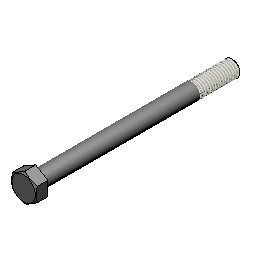
COTS 4 Post Jig v1.00 (Autodesk Fusion 360 archive; units mm, degrees)
design "Hex Bolt ASME B18.2.1 - 1/2-13 UNC x 6 Steel Grade 2 Plain"
description: Hex Bolt ASME B18.2.1 - 1/2-13 UNC x 6
part number: HB ASME B18.2.1 - 1/2-13 UNC x 6 Steel Grade 2 Plain
Autodesk Fusion 360 part; units mm, degrees
sketch "Sketch1" plane through (0, 0, 0) normal (0, 1, 0) x (1, 0, 0)
  line L0 (-6.35, 0) -> (-6.35, 152.4)
  line L1 (-6.35, 152.4) -> (0, 152.4)
  line L2 (0, 152.4) -> (0, -9.2456)
  line L3 (-6.35, 0) -> (-11.0014, 0)
  line L4 (-11.0014, 0) -> (-11.0014, -8.1183)
  line L5 (-9.0487, -9.2456) -> (0, -9.2456)
  line L6 (-11.0014, -8.1183) -> (-9.0487, -9.2456)
  dimension "d81" = 22.0028
  dimension "d135" = 12.7
  dimension "d148" = 9.2456
  dimension "d149" = 152.4
  dimension "d170" = 18.0975
  dimension "d171" = 30
  constraint perpendicular L0 L1
  constraint perpendicular L0 L3
  constraint coincident origin L3
  constraint vertical L0
  constraint vertical L2
  constraint parallel L2 L4
  constraint coincident L2 L5.end
  constraint perpendicular L2 L5
  constraint coincident L0.start L3.start
  constraint coincident L0.end L1.start
  constraint coincident origin L2
  measures "d148" distance of L3 L5
  measures "d149" distance of L1 L3
  measures "d171" angle of L5 L6
revolve "Revolve1" add sketch "Sketch1" angle 360 about axis through (0, 0, -152.4) along (0, 0, 1)
sketch "Sketch8" plane through (0, 0, 9.2456) normal (0, 0, 1) x (1, 0, 0)
  line L0 (0, 0) -> (-9.525, 0) construction
  line L1 (-9.525, -5.505) -> (-9.525, 5.505)
  circle A0 centre (0, 0) radius 11.0014
  dimension "d114" = 9.525
  constraint coincident L0.start A0.centre
  constraint horizontal L0
  constraint perpendicular L0 L1
  constraint coincident L1.end A0
  constraint coincident L0.end L1
  constraint coincident L1.start A0
  measures "d114" distance of L0.start L1
extrude "Extrude5" cut sketch "Sketch8" against normal blind 9.2456 contours L1 A0 picked at (-9.7632, -1.3408)
pattern_circular "C-Pattern2" count 6 over 360 about axis through (0, 0, 1.75) along (0, 0, 1) of "Extrude5"
fillet "Fillet7" radius 0.762 1 edges at (-5.9203, 2.2963, 0)
thread "Thread3" "ANSI Unified Screw Threads 0.5 1/2-13 UNC 1/2-13 UNC 2A" major diameter 12.5247 minor diameter 10.3353 pitch 1.9538 angle 60 resizes the face on face at (-6.3421, 0.3165, -51.308) from (0, 0, -120.65) to (0, 0, -152.4)
sketch "Sketch13" plane through (0, 0, 0) normal (0, 1, 0) x (1, 0, 0)
  line L0 (0, 152.4) -> (0, -9.2456)
  line L1 (0, 152.4) -> (-6.477, 152.4)
  line L2 (-6.477, 152.4) -> (-6.477, 151.2014)
  line L3 (-6.477, 151.2014) -> (-5.1514, 152.4)
  dimension "d172" = 1.1986
  dimension "d173" = 5.1514
  dimension "d174" = 6.477
  constraint coincident L0.start L1.start
  constraint perpendicular L0 L1
  constraint perpendicular L1 L2
  constraint coincident L1 L3.end
  measures "d172" distance of L1 L2.end
  measures "d173" distance of L0 L3.end
  measures "d174" distance of L0.start L2
revolve "Revolve4" cut sketch "Sketch13" angle 360 about axis through (0, 0, 1.75) along (0, 0, 1)
equation "d81 = adsk_headdia"
equation "d89 = -adsk_headh"
equation "d114 = adsk_waflat / 2"
equation "d135 = adsk_nomdia"
equation "adsk_nomlen = 6.00 in"
equation "adsk_headh = 0.364 in"
equation "adsk_headdia = 0.86625 in"
equation "adsk_nomdia = 0.50 in"
equation "adsk_waflat = 0.75 in"
equation "adsk_thrlen = 1.25 in"
equation "adsk_midfillet = 0.03 in"
equation "d148 = adsk_headh"
equation "d149 = adsk_nomlen"
equation "d151 = adsk_midfillet"
equation "adsk_endpointdia = 0.405623 in"
equation "adsk_startlen = 0.047188 in"
equation "d170 = adsk_waflat * 0.95"
equation "d172 = adsk_startlen"
equation "d173 = adsk_endpointdia / 2"
equation "d174 = adsk_nomdia * 0.51"
equation "d176 = min(adsk_thrlen; adsk_nomlen - adsk_midfillet - 0.001 in)"

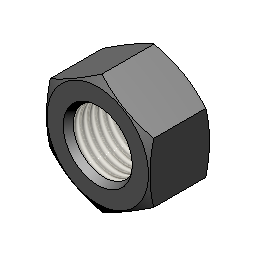
design "Hex Nut ASME B18.2.2 - 3/8-24 Steel Grade 2H Plain"
description: Hex Nut ASME B18.2.2 - 3/8-24
part number: HN ASME B18.2.2 - 3/8-24 Steel Grade 2H Plain
Autodesk Fusion 360 part; units mm, degrees
sketch "Sketch1" plane through (0, 0, 0) normal (0, 1, 0) x (1, 0, 0)
  line L0 (0, 0) -> (0, -8.3566)
  line L1 (-4.7625, 0) -> (-7.0071, 0)
  line L2 (-7.0071, 0) -> (-8.2584, -0.5835)
  line L3 (-8.2584, -0.5835) -> (-8.2584, -7.7731)
  line L4 (-8.2584, -7.7731) -> (-7.0071, -8.3566)
  line L5 (-7.0071, -8.3566) -> (-4.7625, -8.3566)
  line L6 (-4.7625, -8.3566) -> (-4.7625, 0)
  line L7 (-7.0071, -8.3566) -> (-7.0071, 0) construction
  dimension "d121" = 9.525
  dimension "d122" = 25
  dimension "d123" = 25
  dimension "d128" = 16.5167
  dimension "d170" = 14.0142
  dimension "d176" = 8.3566
  constraint vertical L0
  constraint coincident L0 L0.end
  constraint coincident origin L0
  constraint horizontal L1
  constraint perpendicular L1 L3
  constraint perpendicular L3 L5
  constraint perpendicular L5 L6
  constraint coincident L0.start L1
  constraint coincident L0.end L5
  constraint coincident L0.start origin
  constraint vertical L7
  measures "d122" angle of L1 L2
  measures "d123" angle of L4 L5
  measures "d176" distance of L1.start L5
revolve "Revolve1" add sketch "Sketch1" angle 360 about axis through (0, 0, 0) along (0, 0, 1)
sketch "Sketch8" plane through (0, 0, 8.3566) normal (0, 0, 1) x (1, 0, 0)
  line L0 (0, 0) -> (-14.3002, 0) construction
  line L1 (-7.1501, -4.1324) -> (-7.1501, 4.1324)
  circle A0 centre (0, 0) radius 4.7625
  circle A1 centre (0, 0) radius 8.2584
  dimension "d114" = 7.1501
  constraint horizontal L0
  constraint perpendicular L0 L1
  constraint midpoint L0 L1
  constraint coincident L0.start A0.centre
  constraint coincident L1.end A1
  measures "d114" distance of L0.start L1
extrude "Extrude5" cut sketch "Sketch8" against normal blind 8.3566 contours L1 A1 picked at (-7.3289, 1.0065)
pattern_circular "C-Pattern2" count 6 over 360 about axis through (0, 0, 1.75) along (0, 0, 1) of "Extrude5"
thread "Thread3" "ANSI Unified Screw Threads 0.375 3/8-24 UNF 3/8-24 UNF 2B" major diameter 9.525 minor diameter 8.509 pitch 1.0583 angle 60 resizes the face on face at (-4.7388, 0.4742, 2.7855)
sketch "Sketch12" plane through (0, 0, 0) normal (0, 1, 0) x (1, 0, 0)
  line L0 (0, 0) -> (-4.7625, 0)
  line L1 (0, 0) -> (0, -8.3566)
  line L2 (0, -8.3566) -> (-4.7625, -8.3566)
  line L3 (-4.7625, -8.3566) -> (-2.3502, -4.1783)
  line L4 (-4.7625, 0) -> (-2.3502, -4.1783)
  dimension "d164" = 60
  dimension "d165" = 60
  dimension "d175" = 4.7625
  constraint coincident L0.start L1.start
  constraint horizontal L0
  constraint coincident L1.end L2.start
  constraint perpendicular L1 L2
  constraint vertical L0.end L2.end
  constraint coincident L3.end L4.end
  measures "d164" angle of L0 L4
  measures "d165" angle of L2 L3
  measures "d175" distance of L0.end L1
revolve "Revolve3" cut sketch "Sketch12" angle 360 about axis through (0, 0, 1.75) along (0, 0, 1)
equation "d89 = -adsk_nheig"
equation "d114 = adsk_waflat / 2"
equation "adsk_chamang1 = 25.00 deg"
equation "adsk_chamang2 = 25.00 deg"
equation "d121 = adsk_nomdia"
equation "d122 = adsk_chamang1"
equation "d123 = adsk_chamang2"
equation "d128 = adsk_maxdia"
equation "adsk_nheig = 0.329 in"
equation "adsk_maxdia = 0.650265 in"
equation "adsk_nomdia = 0.375 in"
equation "adsk_waflat = 0.563 in"
equation "d162 = adsk_nheig"
equation "adsk_beardia = adsk_waflat * 0.98"
equation "d170 = adsk_beardia"
equation "d175 = adsk_nomdia * 0.50"
equation "d176 = adsk_nheig"

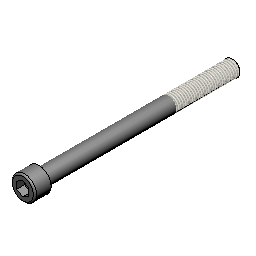
design "Hexagon Socket Head Cap Screw ANSI B18.3 - 1/4-28 UNF x 3 Steel Grade 2 Plain"
description: Hexagon Socket Head Cap Screw ANSI B18.3 - 1/4-28 UNF x 3
part number: HSHCS ANSI B18.3 - 1/4-28 UNF x 3 Steel Grade 2 Plain
Autodesk Fusion 360 part; units mm, degrees
sketch "Sketch1" plane through (0, 0, 0) normal (0, 1, 0) x (1, 0, 0)
  line L0 (-3.175, 0) -> (-3.175, 76.2)
  line L1 (-3.175, 76.2) -> (0, 76.2)
  line L2 (0, 76.2) -> (0, -6.35)
  line L3 (-3.175, 0) -> (-4.7625, 0)
  line L4 (-4.7625, 0) -> (-4.7625, -6.35)
  line L5 (-4.7625, -6.35) -> (0, -6.35)
  dimension "d9" = 6.35
  dimension "d66" = 9.525
  dimension "d107" = 6.35
  dimension "d108" = 76.2
  constraint perpendicular L0 L1
  constraint collinear origin L1.end L2.end
  constraint perpendicular L0 L3
  constraint coincident origin L3
  constraint vertical L0
  constraint vertical L2
  constraint parallel L2 L4
  constraint coincident L2 L5.end
  constraint perpendicular L2 L5
  measures "d107" distance of L3.end L5
  measures "d108" distance of origin L1
revolve "Revolve1" add sketch "Sketch1" angle 360 about axis through (0, 0, -76.2) along (0, 0, 1)
ref_plane "WorkPlane1" through (0, 0, 6.35) normal (0, 0, 1) x (1, 0, 0)
sketch "Sketch6" plane through (0, 0, 6.35) normal (0, 0, 1) x (1, 0, 0)
  line L0 (-2.3876, 0) -> (2.3876, 0) construction
  line L1 (0, 0) -> (-2.3876, 1.3785)
  line L2 (-2.3876, -1.3785) -> (-2.3876, 1.3785)
  line L3 (-2.3876, -1.3785) -> (0, 0)
  dimension "d106" = 150
  dimension "d109" = 4.7752
  constraint horizontal L0
  constraint midpoint L1.start L0
  constraint coincident L1.start L3.end
  constraint perpendicular L0 L2
  constraint midpoint L0.start L2
  constraint coincident L1.end L2.end
  measures "d106" angle of L0 L1
  measures "d109" distance of L0.end L2
extrude "Extrude1" cut sketch "Sketch6" against normal blind 3.048
pattern_circular "C-Pattern1" count 6 over 360 about axis through (0, 0, 1.75) along (0, 0, 1) of "Extrude1"
extrude "Extrude2" cut 1 faces at (0.7959, 0.4595, 3.302) along direction (0, 0, -1) blind 3.048 draft -85
thread "Thread3" "ANSI Unified Screw Threads 0.25 1/4-28 UNF 1/4-28 UNF 2A" major diameter 6.2433 minor diameter 5.2426 pitch 0.9071 angle 60 resizes the face on face at (-3.1711, 0.1583, -50.8) from (0, 0, -50.8) to (0, 0, -76.2)
fillet "Fillet4" radius 0.635 1 edges at (-4.4402, 1.7222, 6.35)
sketch "Sketch7" plane through (0, 0, 0) normal (0, 1, 0) x (1, 0, 0)
  line L0 (-3.2385, 76.2) -> (-3.2385, 75.659)
  line L1 (-3.2385, 75.659) -> (-2.634, 76.2)
  line L2 (0, 76.2) -> (0, -6.35)
  line L3 (-3.2385, 76.2) -> (0, 76.2)
  dimension "d103" = 3.2385
  dimension "d110" = 2.634
  dimension "d111" = 0.541
  constraint coincident L2.start L3.end
  constraint perpendicular L2 L3
  constraint coincident L1.end L3
  constraint perpendicular L0 L3
  measures "d103" distance of origin L0
  measures "d110" distance of L1.end L2
  measures "d111" distance of L0.end L3
revolve "Revolve3" cut sketch "Sketch7" angle 360 about axis through (0, 0, 1.75) along (0, 0, 1)
equation "d9 = adsk_nomdia"
equation "d31 = -adsk_phildepth"
equation "d66 = adsk_headdia"
equation "d71 = adsk_headh"
equation "d76 = -adsk_phildepth"
equation "adsk_nomlen = 3.00 in"
equation "adsk_headh = 0.25 in"
equation "adsk_headdia = 0.375 in"
equation "adsk_nomdia = 0.25 in"
equation "adsk_philwidth = 0.188 in"
equation "adsk_phildepth = 0.12 in"
equation "adsk_thrlen = 1.00 in"
equation "d93 = adsk_nomdia * 0.1"
equation "adsk_startlen = 0.0213 in"
equation "adsk_endpointdia = 0.2074 in"
equation "d103 = adsk_nomdia * 0.51"
equation "d107 = adsk_headh"
equation "d108 = adsk_nomlen"
equation "d109 = adsk_philwidth"
equation "d110 = adsk_endpointdia / 2"
equation "d111 = adsk_startlen"
equation "d113 = min(adsk_thrlen; adsk_nomlen - 0.001 mm)"

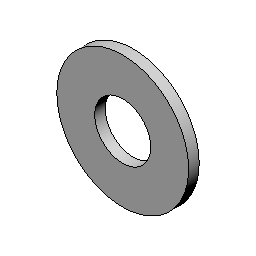
design "Plain Washer ASME B18.21.1 - 1/2 - Regular - Type B Steel 100 HV Zinc"
description: Plain Washer ASME B18.21.1 - 1/2 - Regular - Type B
part number: PW ASME B18.21.1 - 1/2 - BR Steel 100 HV Zinc
Autodesk Fusion 360 part; units mm, degrees
sketch "Sketch1" plane through (0, 0, 0) normal (0, 0, 1) x (1, 0, 0)
  circle A0 centre (0, 0) radius 15.875
  circle A1 centre (0, 0) radius 6.7437
  dimension "d4" = 31.75
  dimension "d5" = 13.4874
  constraint coincident A0.centre A1.centre
  measures "d4" diameter of A0
  measures "d5" diameter of A1
extrude "Extrude2" add sketch "Sketch1" along normal blind 2.54
equation "d4 = adsk_woutdia"
equation "d5 = adsk_windia"
equation "adsk_woutdia = 1.25 in"
equation "adsk_windia = 0.531 in"
equation "adsk_wthick = 0.10 in"
equation "d20 = adsk_wthick"
equation "d41 = adsk_wthick"

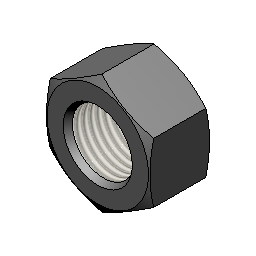
design "Hex Nut ASME B18.2.2 - 1/2-20 Steel Grade 2H Plain"
description: Hex Nut ASME B18.2.2 - 1/2-20
part number: HN ASME B18.2.2 - 1/2-20 Steel Grade 2H Plain
Autodesk Fusion 360 part; units mm, degrees
sketch "Sketch1" plane through (0, 0, 0) normal (0, 1, 0) x (1, 0, 0)
  line L0 (0, 0) -> (0, -11.1252)
  line L1 (-6.35, 0) -> (-9.3345, 0)
  line L2 (-9.3345, 0) -> (-11.0014, -0.7773)
  line L3 (-11.0014, -0.7773) -> (-11.0014, -10.3479)
  line L4 (-11.0014, -10.3479) -> (-9.3345, -11.1252)
  line L5 (-9.3345, -11.1252) -> (-6.35, -11.1252)
  line L6 (-6.35, -11.1252) -> (-6.35, 0)
  line L7 (-9.3345, -11.1252) -> (-9.3345, 0) construction
  dimension "d121" = 12.7
  dimension "d122" = 25
  dimension "d123" = 25
  dimension "d128" = 22.0028
  dimension "d170" = 18.669
  dimension "d176" = 11.1252
  constraint vertical L0
  constraint coincident L0 L0.end
  constraint coincident origin L0
  constraint horizontal L1
  constraint perpendicular L1 L3
  constraint perpendicular L3 L5
  constraint perpendicular L5 L6
  constraint coincident L0.start L1
  constraint coincident L0.end L5
  constraint coincident L0.start origin
  constraint vertical L7
  measures "d122" angle of L1 L2
  measures "d123" angle of L4 L5
  measures "d176" distance of L1.start L5
revolve "Revolve1" add sketch "Sketch1" angle 360 about axis through (0, 0, 0) along (0, 0, 1)
sketch "Sketch8" plane through (0, 0, 11.1252) normal (0, 0, 1) x (1, 0, 0)
  line L0 (0, 0) -> (-19.05, 0) construction
  line L1 (-9.525, -5.505) -> (-9.525, 5.505)
  circle A0 centre (0, 0) radius 6.35
  circle A1 centre (0, 0) radius 11.0014
  dimension "d114" = 9.525
  constraint horizontal L0
  constraint perpendicular L0 L1
  constraint midpoint L0 L1
  constraint coincident L0.start A0.centre
  constraint coincident L1.end A1
  measures "d114" distance of L0.start L1
extrude "Extrude5" cut sketch "Sketch8" against normal blind 11.1252 contours L1 A1 picked at (-9.7632, 1.3408)
pattern_circular "C-Pattern2" count 6 over 360 about axis through (0, 0, 1.75) along (0, 0, 1) of "Extrude5"
thread "Thread3" "ANSI Unified Screw Threads 0.5 1/2-20 UNF 1/2-20 UNF 2B" major diameter 12.7 minor diameter 11.4681 pitch 1.27 angle 60 resizes the face on face at (-6.3421, 0.3165, 7.4168)
sketch "Sketch12" plane through (0, 0, 0) normal (0, 1, 0) x (1, 0, 0)
  line L0 (0, 0) -> (-6.35, 0)
  line L1 (0, 0) -> (0, -11.1252)
  line L2 (0, -11.1252) -> (-6.35, -11.1252)
  line L3 (-6.35, -11.1252) -> (-3.1384, -5.5626)
  line L4 (-6.35, 0) -> (-3.1384, -5.5626)
  dimension "d164" = 60
  dimension "d165" = 60
  dimension "d175" = 6.35
  constraint coincident L0.start L1.start
  constraint horizontal L0
  constraint coincident L1.end L2.start
  constraint perpendicular L1 L2
  constraint vertical L0.end L2.end
  constraint coincident L3.end L4.end
  measures "d164" angle of L0 L4
  measures "d165" angle of L2 L3
  measures "d175" distance of L0.end L1
revolve "Revolve3" cut sketch "Sketch12" angle 360 about axis through (0, 0, 1.75) along (0, 0, 1)
equation "d89 = -adsk_nheig"
equation "d114 = adsk_waflat / 2"
equation "adsk_chamang1 = 25.00 deg"
equation "adsk_chamang2 = 25.00 deg"
equation "d121 = adsk_nomdia"
equation "d122 = adsk_chamang1"
equation "d123 = adsk_chamang2"
equation "d128 = adsk_maxdia"
equation "adsk_nheig = 0.438 in"
equation "adsk_maxdia = 0.86625 in"
equation "adsk_nomdia = 0.50 in"
equation "adsk_waflat = 0.75 in"
equation "d162 = adsk_nheig"
equation "adsk_beardia = adsk_waflat * 0.98"
equation "d170 = adsk_beardia"
equation "d175 = adsk_nomdia * 0.50"
equation "d176 = adsk_nheig"

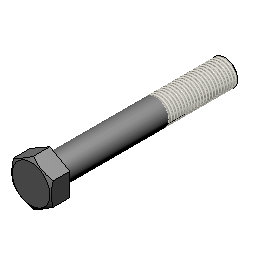
design "Hex Bolt ANSI B18.2.1 - 3/8-24 UNF x 2.5 Steel Grade 2 Plain"
description: Hex Bolt ANSI B18.2.1 - 3/8-24 UNF x 2.5
part number: HB ANSI B18.2.1 - 3/8-24 UNF x 2.5 Steel Grade 2 Plain
Autodesk Fusion 360 part; units mm, degrees
sketch "Sketch1" plane through (0, 0, 0) normal (0, 1, 0) x (1, 0, 0)
  line L0 (-4.7625, 0) -> (-4.7625, 63.5)
  line L1 (-4.7625, 63.5) -> (0, 63.5)
  line L2 (0, 63.5) -> (0, -6.8072)
  line L3 (-4.7625, 0) -> (-8.2437, 0)
  line L4 (-8.2437, 0) -> (-8.2437, -5.9624)
  line L5 (-6.7805, -6.8072) -> (0, -6.8072)
  line L6 (-8.2437, -5.9624) -> (-6.7805, -6.8072)
  dimension "d81" = 16.4874
  dimension "d135" = 9.525
  dimension "d148" = 6.8072
  dimension "d149" = 63.5
  dimension "d170" = 13.5611
  dimension "d171" = 30
  constraint perpendicular L0 L1
  constraint perpendicular L0 L3
  constraint coincident origin L3
  constraint vertical L0
  constraint vertical L2
  constraint parallel L2 L4
  constraint coincident L2 L5.end
  constraint perpendicular L2 L5
  constraint coincident L0.start L3.start
  constraint coincident L0.end L1.start
  constraint coincident origin L2
  measures "d148" distance of L3 L5
  measures "d149" distance of L1 L3
  measures "d171" angle of L5 L6
revolve "Revolve1" add sketch "Sketch1" angle 360 about axis through (0, 0, -63.5) along (0, 0, 1)
sketch "Sketch8" plane through (0, 0, 6.8072) normal (0, 0, 1) x (1, 0, 0)
  line L0 (0, 0) -> (-7.1374, 0) construction
  line L1 (-7.1374, -4.1251) -> (-7.1374, 4.1251)
  circle A0 centre (0, 0) radius 8.2437
  dimension "d114" = 7.1374
  constraint coincident L0.start A0.centre
  constraint horizontal L0
  constraint perpendicular L0 L1
  constraint coincident L1.end A0
  constraint coincident L0.end L1
  constraint coincident L1.start A0
  measures "d114" distance of L0.start L1
extrude "Extrude5" cut sketch "Sketch8" against normal blind 6.8072 contours L1 A0 picked at (-7.3159, 1.0047)
pattern_circular "C-Pattern2" count 6 over 360 about axis through (0, 0, 1.75) along (0, 0, 1) of "Extrude5"
fillet "Fillet7" radius 0.762 1 edges at (-4.4402, 1.7222, 0)
thread "Thread3" "ANSI Unified Screw Threads 0.375 3/8-24 UNF 3/8-24 UNF 2A" major diameter 9.4056 minor diameter 8.2372 pitch 1.0583 angle 60 resizes the face on face at (-4.7566, 0.2374, -21.6747) from (0, 0, -38.1) to (0, 0, -63.5)
sketch "Sketch13" plane through (0, 0, 0) normal (0, 1, 0) x (1, 0, 0)
  line L0 (0, 63.5) -> (0, -6.8072)
  line L1 (0, 63.5) -> (-4.8577, 63.5)
  line L2 (-4.8577, 63.5) -> (-4.8577, 62.8508)
  line L3 (-4.8577, 62.8508) -> (-4.1133, 63.5)
  dimension "d172" = 0.6492
  dimension "d173" = 4.1133
  dimension "d174" = 4.8578
  constraint coincident L0.start L1.start
  constraint perpendicular L0 L1
  constraint perpendicular L1 L2
  constraint coincident L1 L3.end
  measures "d172" distance of L1 L2.end
  measures "d173" distance of L0 L3.end
  measures "d174" distance of L0.start L2
revolve "Revolve4" cut sketch "Sketch13" angle 360 about axis through (0, 0, 1.75) along (0, 0, 1)
equation "d81 = adsk_headdia"
equation "d89 = -adsk_headh"
equation "d114 = adsk_waflat / 2"
equation "d135 = adsk_nomdia"
equation "adsk_nomlen = 2.50 in"
equation "adsk_headh = 0.268 in"
equation "adsk_headdia = 0.64911 in"
equation "adsk_nomdia = 0.375 in"
equation "adsk_waflat = 0.562 in"
equation "adsk_thrlen = 1.00 in"
equation "adsk_midfillet = 0.03 in"
equation "d148 = adsk_headh"
equation "d149 = adsk_nomlen"
equation "d151 = adsk_midfillet"
equation "adsk_endpointdia = 0.323879 in"
equation "adsk_startlen = 0.025561 in"
equation "d170 = adsk_waflat * 0.95"
equation "d172 = adsk_startlen"
equation "d173 = adsk_endpointdia / 2"
equation "d174 = adsk_nomdia * 0.51"
equation "d176 = min(adsk_thrlen; adsk_nomlen - adsk_midfillet - 0.001 in)"

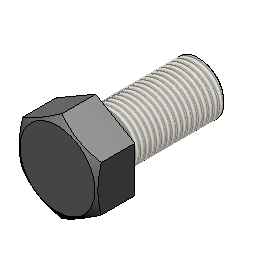
design "Hex Bolt ANSI B18.2.1 - 1/2-20 UNF x 1 Steel Grade 2 Plain"
description: Hex Bolt ANSI B18.2.1 - 1/2-20 UNF x 1
part number: HB ANSI B18.2.1 - 1/2-20 UNF x 1 Steel Grade 2 Plain
Autodesk Fusion 360 part; units mm, degrees
sketch "Sketch1" plane through (0, 0, 0) normal (0, 1, 0) x (1, 0, 0)
  line L0 (-6.35, 0) -> (-6.35, 25.4)
  line L1 (-6.35, 25.4) -> (0, 25.4)
  line L2 (0, 25.4) -> (0, -9.2456)
  line L3 (-6.35, 0) -> (-11.0014, 0)
  line L4 (-11.0014, 0) -> (-11.0014, -8.1183)
  line L5 (-9.0487, -9.2456) -> (0, -9.2456)
  line L6 (-11.0014, -8.1183) -> (-9.0487, -9.2456)
  dimension "d81" = 22.0028
  dimension "d135" = 12.7
  dimension "d148" = 9.2456
  dimension "d149" = 25.4
  dimension "d170" = 18.0975
  dimension "d171" = 30
  constraint perpendicular L0 L1
  constraint perpendicular L0 L3
  constraint coincident origin L3
  constraint vertical L0
  constraint vertical L2
  constraint parallel L2 L4
  constraint coincident L2 L5.end
  constraint perpendicular L2 L5
  constraint coincident L0.start L3.start
  constraint coincident L0.end L1.start
  constraint coincident origin L2
  measures "d148" distance of L3 L5
  measures "d149" distance of L1 L3
  measures "d171" angle of L5 L6
revolve "Revolve1" add sketch "Sketch1" angle 360 about axis through (0, 0, -25.4) along (0, 0, 1)
sketch "Sketch8" plane through (0, 0, 9.2456) normal (0, 0, 1) x (1, 0, 0)
  line L0 (0, 0) -> (-9.525, 0) construction
  line L1 (-9.525, -5.505) -> (-9.525, 5.505)
  circle A0 centre (0, 0) radius 11.0014
  dimension "d114" = 9.525
  constraint coincident L0.start A0.centre
  constraint horizontal L0
  constraint perpendicular L0 L1
  constraint coincident L1.end A0
  constraint coincident L0.end L1
  constraint coincident L1.start A0
  measures "d114" distance of L0.start L1
extrude "Extrude5" cut sketch "Sketch8" against normal blind 9.2456 contours L1 A0 picked at (-9.7632, 1.3408)
pattern_circular "C-Pattern2" count 6 over 360 about axis through (0, 0, 1.75) along (0, 0, 1) of "Extrude5"
fillet "Fillet7" radius 0.762 1 edges at (-5.9203, 2.2963, 0)
thread "Thread3" "ANSI Unified Screw Threads 0.5 1/2-20 UNF 1/2-20 UNF 2A" major diameter 12.5654 minor diameter 11.1557 pitch 1.27 angle 60 resizes the face on face at (-6.3421, 0.3165, -8.9747) from (0, 0, -3.175) to (0, 0, -25.4)
sketch "Sketch13" plane through (0, 0, 0) normal (0, 1, 0) x (1, 0, 0)
  line L0 (0, 25.4) -> (0, -9.2456)
  line L1 (0, 25.4) -> (-6.477, 25.4)
  line L2 (-6.477, 25.4) -> (-6.477, 24.6209)
  line L3 (-6.477, 24.6209) -> (-5.5709, 25.4)
  dimension "d172" = 0.7791
  dimension "d173" = 5.5709
  dimension "d174" = 6.477
  constraint coincident L0.start L1.start
  constraint perpendicular L0 L1
  constraint perpendicular L1 L2
  constraint coincident L1 L3.end
  measures "d172" distance of L1 L2.end
  measures "d173" distance of L0 L3.end
  measures "d174" distance of L0.start L2
revolve "Revolve4" cut sketch "Sketch13" angle 360 about axis through (0, 0, 1.75) along (0, 0, 1)
equation "d81 = adsk_headdia"
equation "d89 = -adsk_headh"
equation "d114 = adsk_waflat / 2"
equation "d135 = adsk_nomdia"
equation "adsk_nomlen = 1.00 in"
equation "adsk_headh = 0.364 in"
equation "adsk_headdia = 0.86625 in"
equation "adsk_nomdia = 0.50 in"
equation "adsk_waflat = 0.75 in"
equation "adsk_thrlen = 0.875 in"
equation "adsk_midfillet = 0.03 in"
equation "d148 = adsk_headh"
equation "d149 = adsk_nomlen"
equation "d151 = adsk_midfillet"
equation "adsk_endpointdia = 0.438655 in"
equation "adsk_startlen = 0.030673 in"
equation "d170 = adsk_waflat * 0.95"
equation "d172 = adsk_startlen"
equation "d173 = adsk_endpointdia / 2"
equation "d174 = adsk_nomdia * 0.51"
equation "d176 = min(adsk_thrlen; adsk_nomlen - adsk_midfillet - 0.001 in)"

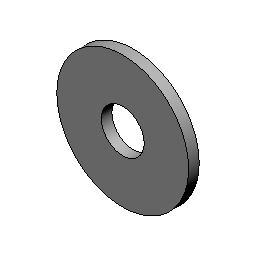
design "Plain Washer ANSI B18.22.1 - 3/8 - Wide - Type B Steel 100 HV Plain"
description: Plain Washer ANSI B18.22.1 - 3/8 - Wide - Type B
part number: PW ANSI B18.22.1 - 3/8 - BW Steel 100 HV Plain
Autodesk Fusion 360 part; units mm, degrees
sketch "Sketch1" plane through (0, 0, 0) normal (0, 0, 1) x (1, 0, 0)
  circle A0 centre (0, 0) radius 15.875
  circle A1 centre (0, 0) radius 5.1562
  dimension "d4" = 31.75
  dimension "d5" = 10.3124
  constraint coincident A0.centre A1.centre
  measures "d4" diameter of A0
  measures "d5" diameter of A1
extrude "Extrude2" add sketch "Sketch1" along normal blind 2.54
equation "d4 = adsk_woutdia"
equation "d5 = adsk_windia"
equation "adsk_woutdia = 1.25 in"
equation "adsk_windia = 0.406 in"
equation "adsk_wthick = 0.10 in"
equation "d20 = adsk_wthick"
equation "d41 = adsk_wthick"
